Autodesk Fusion 360 part; units mm, degrees
note: some values were not read from the file. Chosen so that the rebuilt part matches the saved one: which face or edge a step refers to; which pieces of a blend or face edit are solid.
(part 2 of 2)
sketch "Sketch12" plane through (0, 0, 7.8) normal (0, 0, -1) x (1, 0, 0) in component "Cover"
  line L0 (18.796, -18.1343) -> (28.396, -18.1343)
  line L1 (28.396, -18.1343) -> (28.396, -17.465)
  line L2 (28.396, -17.465) -> (23.596, -17.465)
  arc A0 (23.596, -12.265) -> (23.596, -17.465) centre (23.596, -14.865) ccw
  line L3 (23.596, -12.265) -> (28.396, -12.265)
  line L4 (28.396, -12.265) -> (28.396, -1.3173)
  arc A1 (28.396, -1.3173) -> (26.826, 0.2527) centre (26.826, -1.3173) ccw
  line L5 (26.826, 0.2527) -> (7.1, 0.2527)
  line L6 (7.1, 0.2527) -> (7.1, -3.5473)
  arc A2 (4.5, -6.1473) -> (7.1, -3.5473) centre (4.5, -3.5473) ccw
  line L7 (4.5, -6.1473) -> (-0.3, -6.1473)
  line L8 (-0.3, -6.1473) -> (-0.3, -7.1473)
  line L9 (-0.3, -7.1473) -> (-0.3, -21.5343)
  line L10 (-0.3, -21.5343) -> (-0.3, -23.9343)
  line L11 (-0.3, -23.9343) -> (4.5, -23.9343)
  arc A3 (7.1, -26.5343) -> (4.5, -23.9343) centre (4.5, -26.5343) ccw
  line L12 (7.1, -26.5343) -> (7.1, -30.1343)
  line L13 (7.1, -30.1343) -> (26.826, -30.1343)
  arc A4 (26.826, -30.1343) -> (28.2889, -29.1343) centre (26.826, -28.5643) ccw
  line L14 (28.2889, -29.1343) -> (18.796, -29.1343)
  line L15 (18.796, -29.1343) -> (18.796, -18.1343)
  line L16 (-0.3, -21.5343) -> (11.7, -21.5343)
  line L17 (11.7, -21.5343) -> (11.7, -7.1473)
  line L18 (11.7, -7.1473) -> (-0.3, -7.1473)
  dimension "d113" = 12
  constraint coincident L9.end L10.start
  constraint perpendicular L9 L16
  constraint perpendicular L16 L17
  constraint perpendicular L9 L18
  constraint coincident L8.end L9.start
  measures "d113" distance of L9 L17
extrude "Extrude11'" cut sketch "Sketch12" against normal through all contours L9 L16 L17 L18 bodies 3 in component "Cover"
sketch "Sketch13" plane through (0, 0, 7.8) normal (0, 0, -1) x (1, 0, 0) in component "Cover"
  line L0 (11.7, -21.5343) -> (-0.3, -21.5343)
  line L1 (-0.3, -21.5343) -> (-0.3, -23.9343)
  line L2 (-0.3, -23.9343) -> (4.5, -23.9343)
  arc A0 (7.1, -26.5343) -> (4.5, -23.9343) centre (4.5, -26.5343) ccw
  line L3 (7.1, -26.5343) -> (7.1, -30.1343)
  line L4 (7.1, -30.1343) -> (26.826, -30.1343)
  arc A1 (26.826, -30.1343) -> (28.2889, -29.1343) centre (26.826, -28.5643) ccw
  line L5 (28.2889, -29.1343) -> (18.796, -29.1343)
  line L6 (18.796, -29.1343) -> (18.796, -18.1343)
  line L7 (18.796, -18.1343) -> (28.396, -18.1343)
  line L8 (28.396, -18.1343) -> (28.396, -17.465)
  line L9 (28.396, -17.465) -> (23.596, -17.465)
  arc A2 (23.596, -12.265) -> (23.596, -17.465) centre (23.596, -14.865) ccw
  line L10 (23.596, -12.265) -> (28.396, -12.265)
  line L11 (28.396, -12.265) -> (28.396, -1.3173)
  arc A3 (28.396, -1.3173) -> (26.826, 0.2527) centre (26.826, -1.3173) ccw
  line L12 (26.826, 0.2527) -> (7.1, 0.2527)
  line L13 (7.1, 0.2527) -> (7.1, -3.5473)
  arc A4 (4.5, -6.1473) -> (7.1, -3.5473) centre (4.5, -3.5473) ccw
  line L14 (4.5, -6.1473) -> (-0.3, -6.1473)
  line L15 (-0.3, -6.1473) -> (-0.3, -7.1473)
  line L16 (-0.3, -7.1473) -> (11.7, -7.1473)
  line L17 (11.7, -7.1473) -> (11.7, -21.5343)
  line L18 (11.7, -18.7408) -> (14.7, -18.7408)
  line L19 (14.7, -18.7408) -> (14.7, -9.9408)
  line L20 (14.7, -9.9408) -> (11.7, -9.9408)
  line L21 (14.7, -14.3408) -> (11.7, -14.3408) construction
  dimension "d115" = 8.8
  dimension "d116" = 3
  constraint coincident L17 L18.start
  constraint perpendicular L17 L18
  constraint perpendicular L18 L19
  constraint coincident L17 L20.end
  constraint perpendicular L17 L20
  constraint midpoint L19 L21.start
  constraint perpendicular L19 L21
  constraint midpoint L17 L21.end
  measures "d115" distance of L18.end L19.end
  measures "d116" distance of L18.start L18.end
extrude "Extrude12'" cut sketch "Sketch13" against normal up to surface (1.6 mm away) contours L17 L18 L19 L20 bodies 3 in component "Cover"
sketch "Sketch15" plane through (0, 0, 7.8) normal (0, 0, -1) x (1, 0, 0) in component "Cover"
  line L0 (14.7, -18.7408) -> (11.7, -18.7408)
  line L1 (11.7, -18.7408) -> (11.7, -21.5343)
  line L2 (11.7, -21.5343) -> (-0.3, -21.5343)
  line L3 (-0.3, -21.5343) -> (-0.3, -23.9343)
  line L4 (-0.3, -23.9343) -> (4.5, -23.9343)
  arc A0 (7.1, -26.5343) -> (4.5, -23.9343) centre (4.5, -26.5343) ccw
  line L5 (7.1, -26.5343) -> (7.1, -30.1343)
  line L6 (7.1, -30.1343) -> (26.826, -30.1343)
  arc A1 (26.826, -30.1343) -> (28.2889, -29.1343) centre (26.826, -28.5643) ccw
  line L7 (28.2889, -29.1343) -> (18.796, -29.1343)
  line L8 (18.796, -29.1343) -> (18.796, -18.1343)
  line L9 (18.796, -18.1343) -> (28.396, -18.1343)
  line L10 (28.396, -18.1343) -> (28.396, -17.465)
  line L11 (28.396, -17.465) -> (23.596, -17.465)
  arc A2 (23.596, -12.265) -> (23.596, -17.465) centre (23.596, -14.865) ccw
  line L12 (23.596, -12.265) -> (28.396, -12.265)
  line L13 (28.396, -12.265) -> (28.396, -1.3173)
  arc A3 (28.396, -1.3173) -> (26.826, 0.2527) centre (26.826, -1.3173) ccw
  line L14 (26.826, 0.2527) -> (7.1, 0.2527)
  line L15 (7.1, 0.2527) -> (7.1, -3.5473)
  arc A4 (4.5, -6.1473) -> (7.1, -3.5473) centre (4.5, -3.5473) ccw
  line L16 (4.5, -6.1473) -> (-0.3, -6.1473)
  line L17 (-0.3, -6.1473) -> (-0.3, -7.1473)
  line L18 (-0.3, -7.1473) -> (11.7, -7.1473)
  line L19 (11.7, -7.1473) -> (11.7, -9.9408)
  line L20 (11.7, -9.9408) -> (14.7, -9.9408)
  line L21 (14.7, -9.9408) -> (14.7, -18.7408)
  line L22 (18.796, -29.1343) -> (18.796, -30.1343)
  constraint coincident L7.end L8.start
  constraint coincident L6 L22.end
  constraint perpendicular L6 L22
extrude "Extrude14" cut sketch "Sketch15" against normal blind 1 contours L6 A1 L7 L22 bodies 3 in component "Cover"
chamfer "Chamfer3" [suppressed] in component "Mount"
component "PCB" placed x (1, 0, 0) y (0, 1, 0) z (0, 0, 1) at (0, 0, 0)
component "Mount" placed x (1, 0, 0) y (0, 1, 0) z (0, 0, 1) at (0, 0, 0)
component "Cover" placed x (1, 0, 0) y (0, 1, 0) z (0, 0, 1) at (0, 0, 0)
equation "d31 = 3.3 mm + 1.5 mm"
equation "d39 = 1.27 mm + 1.5 mm"
